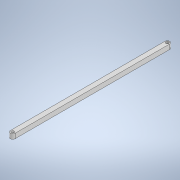
# Autodesk Inventor part: Балка рулевого управления
Saved by Autodesk Inventor 2020 (Build 240168000, 168)
## iProperties
Created: 2021-03-21
Part Number: Балка рулевого управления
Material: Типовые
Document SubType Name: Modeling
Designer: Антон
Density: 1 g/cm^3
Appearance: По умолчанию
Author: Антон
Autodesk Inventor part; units mm, degrees
ref_plane "YZ Plane" through (0, 0, 0) normal (1, 0, 0) x (0, 1, 0)
ref_plane "XZ Plane" through (0, 0, 0) normal (0, 1, 0) x (-1, 0, 0)
ref_plane "XY Plane" through (0, 0, 0) normal (0, 0, 1) x (1, 0, 0)
sketch "Эскиз1" plane through (0, 0, 0) normal (0, 1, 0) x (-1, 0, 0)
  line L0 (0, 0) -> (5, 0)
  line L1 (5, 0) -> (5, -84)
  line L2 (5, -84) -> (0, -84)
  line L3 (0, -84) -> (0, 0)
  line L4 (2.5, 0) -> (2.5, -2.5)
  circle A0 centre (2.5, -2.5) radius 1.5
  dimension "d0" = 5
  dimension "d1" = 84
  dimension "d4" = 2.5
  dimension "d5" = 3
  constraints: 10 end point, 2 parallel, 1 centre point, 1 coincident, 1 horizontal, 1 midpoint, 1 perpendicular, 1 vertical
  measures "d0" distance of L1.end L2.end
  measures "d1" distance of L0.end L1.end
  measures "d4" distance of L4.start L4.end
  measures "d5" diameter of A0
extrude "Выдавливание1" add sketch "Эскиз1" along normal blind 5
fillet "Сопряжение1" radius 2.5 2 edges at (0, 2.5, 0) (-5, 2.5, 0)
mirror "Зеркальное отражение1" about plane through (0, 0, -84) normal (0, 0, -1)
